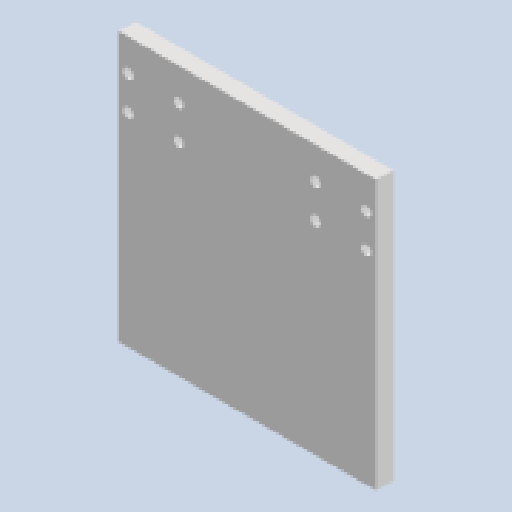
# Autodesk Inventor part: деталь которая двигает
Saved by Autodesk Inventor 2024.2 (Build 282272000, 272)
## iProperties
Created: 2025-11-27
Part Number: деталь которая двигает
Material: Типовые
Document SubType Name: Modeling
Designer: katya_notebook
Density: 1 g/cm^3
Appearance: По умолчанию
Author: katya_notebook
Autodesk Inventor part; units mm, degrees
ref_plane "YZ Plane" through (0, 0, 0) normal (1, 0, 0) x (0, 1, 0)
ref_plane "XZ Plane" through (0, 0, 0) normal (0, 1, 0) x (-1, 0, 0)
ref_plane "XY Plane" through (0, 0, 0) normal (0, 0, 1) x (1, 0, 0)
ref_plane "РабПлоскость1" through (60.4859, 14.4075, 5.5) normal (0, 0, 1) x (1, 0, 0)
sketch "Эскиз1" plane through (60.4859, 14.4075, 5.5) normal (0, 0, 1) x (1, 0, 0)
  line L0 (-8.3, 0) -> (-8.3, -13.5) projected
  line L1 (8.3, -13.5) -> (8.3, 0) projected
  line L2 (36.3, 0) -> (36.3, -13.5) projected
  line L3 (52.9, -13.5) -> (52.9, 0) projected
  line L4 (36.1, -13.5) -> (36.1, -17.1) projected
  line L5 (53.1, -17.1) -> (53.1, -13.5) projected
  line L6 (36.1, -13.5) -> (36.1, 0) projected
  line L7 (53.1, 0) -> (53.1, -13.5) projected
  line L8 (-3.7, 0) -> (-8.3, 0) projected
  line L9 (-8.3, 0) -> (-8.3, -13.5) projected
  line L10 (-3.7, -13.5) -> (-8.3, -13.5) projected
  line L11 (-3.7, -13.5) -> (-3.7, 0) projected
  circle A0 centre (-6, -2.75) radius 1.2 projected
  circle A1 centre (-6, -10.75) radius 1.2 projected
  circle A2 centre (6, -2.75) radius 1.2 projected
  line L12 (8.3, 0) -> (3.7, 0) projected
  line L13 (3.7, 0) -> (3.7, -13.5) projected
  line L14 (8.3, -13.5) -> (3.7, -13.5) projected
  line L15 (8.3, -13.5) -> (8.3, 0) projected
  circle A3 centre (6, -2.75) radius 1.2 projected
  circle A4 centre (6, -10.75) radius 1.2 projected
  line L16 (40.9, 0) -> (36.3, 0) projected
  line L17 (36.3, 0) -> (36.3, -13.5) projected
  line L18 (40.9, -13.5) -> (36.3, -13.5) projected
  line L19 (40.9, -13.5) -> (40.9, 0) projected
  circle A5 centre (38.6, -2.75) radius 1.2 projected
  circle A6 centre (38.6, -10.75) radius 1.2 projected
  line L20 (52.9, 0) -> (48.3, 0) projected
  line L21 (48.3, 0) -> (48.3, -13.5) projected
  line L22 (52.9, -13.5) -> (48.3, -13.5) projected
  line L23 (52.9, -13.5) -> (52.9, 0) projected
  circle A7 centre (50.6, -2.75) radius 1.2 projected
  circle A8 centre (50.6, -10.75) radius 1.2 projected
  line L24 (-8.1442, 4.8798) -> (53.1, 4.8798)
  line L25 (53.1, 4.8798) -> (53.1, -59.1202)
  line L26 (53.1, -59.1202) -> (-8.1442, -59.1202)
  line L27 (-8.1442, -59.1202) -> (-8.1442, 4.8798)
  point P0 (-60.4859, -14.4075)
  dimension "d0" = 64
  constraints: 8 end point, 2 parallel, 1 horizontal, 1 perpendicular
  measures "d0" distance of L24.end L25.end
extrude "Выдавливание1" add sketch "Эскиз1" along normal blind 4 contours L27 L24 L25 L7 L5 L26 L10 L11 L8 | L8 L11 L10 L27 | L14 L13 L12 L1 | L16 L19 L18 L2 | L22 L21 L20 L3
